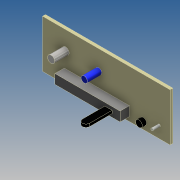
# Autodesk Inventor part: Targeta electrica
Saved by Autodesk Inventor 2016 (Build 200138000, 138)
## iProperties
Created: 2016-05-25
Part Number: Targeta electrica
Material: Polypropylene
Document SubType Name: Modeling
Designer: Familia
Density: 0.899 g/cm^3
Appearance: Smooth - Ash
Author: Familia
Autodesk Inventor part; units mm, degrees
ref_plane "YZ Plane" through (0, 0, 0) normal (1, 0, 0) x (0, 1, 0)
ref_plane "XZ Plane" through (0, 0, 0) normal (0, 1, 0) x (-1, 0, 0)
ref_plane "XY Plane" through (0, 0, 0) normal (0, 0, 1) x (1, 0, 0)
sketch "Sketch1" plane through (0, 0, 0) normal (0, 1, 0) x (-1, 0, 0)
  line L0 (-44, -16.5) -> (44, -16.5)
  line L1 (44, -16.5) -> (44, 16.5)
  line L2 (44, 16.5) -> (-44, 16.5)
  line L3 (-44, 16.5) -> (-44, -16.5)
  line L4 (-44, -16.5) -> (44, 16.5) construction
  line L5 (44, -16.5) -> (-44, 16.5) construction
  point P0 (0, 0)
  dimension "d0" = 33
  dimension "d1" = 88
  constraints: 12 end point, 2 midpoint, 2 parallel, 1 horizontal, 1 perpendicular
  measures "d0" distance of L0.end L1.end
  measures "d1" distance of L1.end L2.end
extrude "Extrusion1" add sketch "Sketch1" along normal blind 2
sketch "Sketch2" plane through (0, 0, 0) normal (0, -1, 0) x (1, 0, 0)
  line L0 (-29, -13.5) -> (16, -13.5)
  line L1 (16, -13.5) -> (16, -7)
  line L2 (16, -7) -> (-29, -7)
  line L3 (-29, -7) -> (-29, -13.5)
  line L4 (44, -16.5) -> (-44, -16.5) projected
  line L5 (-44, -16.5) -> (-44, 16.5) projected
  point P0 (0, 0)
  dimension "d4" = 15
  dimension "d5" = 9.5
  dimension "d6" = 45
  dimension "d7" = 3
  constraints: 8 end point, 2 parallel, 1 horizontal, 1 perpendicular
  measures "d4" distance between parallel lines of L3 L5
  measures "d5" distance between parallel lines of L4 L2
  measures "d6" distance of L1.end L2.end
  measures "d7" distance between parallel lines of L4 L0
extrude "Extrusion2" add sketch "Sketch2" along normal blind 6.5
sketch "Sketch3" plane through (0, -6.5, 0) normal (0, -1, 0) x (1, 0, 0)
  line L0 (5.5, -9.25) -> (10.5, -9.25)
  line L1 (10.5, -9.25) -> (10.5, -11.25)
  line L2 (10.5, -11.25) -> (5.5, -11.25)
  line L3 (5.5, -11.25) -> (5.5, -9.25)
  line L4 (-29, -13.5) -> (16, -13.5) construction
  line L5 (-29, -7) -> (-29, -13.5) construction
  line L6 (-29, -10.25) -> (5.5, -10.25)
  point P0 (0, 0)
  dimension "d10" = 34.5
  dimension "d11" = 5
  dimension "d12" = 2
  constraints: 10 end point, 2 horizontal, 2 midpoint, 2 parallel, 1 perpendicular
  measures "d10" distance of L6.start L6.end
  measures "d11" distance of L0.start L0.end
  measures "d12" distance of L0.end L1.end
extrude "Extrusion3" add sketch "Sketch3" along normal blind 18
full round fillet "Fillet1" first side at (10.5, -12.5, -9.9167) centre faces at (7.1667, -24.5, -9.9167) second side at (5.5, -12.5, -10.5833)
sketch "Sketch4" plane through (0, 0, 0) normal (0, -1, 0) x (1, 0, 0)
  circle A0 centre (-28.0877, 3.7225) radius 2.4593
  circle A1 centre (-5.2453, 3.0457) radius 2.1352
  circle A2 centre (25.5496, -11.5058) radius 2.2905
  circle A3 centre (36.5478, -8.4601) radius 0.8275
  point P0 (0, 0)
  constraints: 4 centre point
extrude "Extrusion4" add sketch "Sketch4" along normal blind 10 contours A0
extrude "Extrusion5" add sketch "Sketch4" along normal blind 10 contours A1
extrude "Extrusion6" add sketch "Sketch4" along normal blind 3 contours A2
extrude "Extrusion7" add sketch "Sketch4" along normal blind 5 contours A3
body "Solid1"
